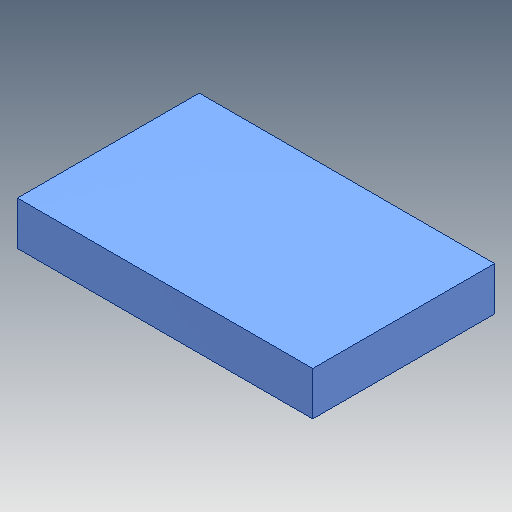
# Autodesk Inventor part: SELECT
Saved by Autodesk Inventor 2017 (Build 210142000, 142)
## iProperties
Part Number: SELECT
Material: Generisch
Document SubType Name: Modeling
Designer: Werkstatt
Density: 1 g/cm^3
Appearance: SWITCH-SPST-SMD-A, SELECT
Author: Werkstatt
Autodesk Inventor part; units mm, degrees
ref_plane "YZ Plane" through (0, 0, 0) normal (1, 0, 0) x (0, 1, 0)
ref_plane "XZ Plane" through (0, 0, 0) normal (0, 1, 0) x (-1, 0, 0)
ref_plane "XY Plane" through (0, 0, 0) normal (0, 0, 1) x (1, 0, 0)
sketch "SWITCH-SPST-SMD-A, SELECT_49" plane through (0, 0, 0) normal (0, 0, 1) x (1, 0, 0)
  line L0 (-3.4135, 2.8) -> (3.35, 2.8)
  line L1 (3.35, 2.8) -> (3.35, -1.3635)
  line L2 (3.35, -1.3635) -> (-3.4135, -1.3635)
  line L3 (-3.4135, -1.3635) -> (-3.4135, 2.8)
  constraints: 8 end point
extrude "Extrusion1" add sketch "SWITCH-SPST-SMD-A, SELECT_49" along normal blind 1
